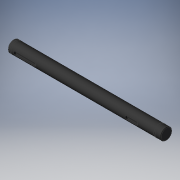
# Autodesk Inventor part: NSFMKRRA10-131-F3-S6-KA5-A19-KB100.5-B11_s
Saved by Autodesk Inventor 2019 (Build 230136000, 136)
## iProperties
Created: 2022-11-16
Part Number: NSFMKRRA10-131-F3-S6-KA5-A19-KB100.5-B11_s
Material: Generic
Catalog Web Link: www.cadenas.de
Description: NSFMKRR, SFMKRR, PSFMKRR, SSFMKRR, NSFHKRR, SFHKRR, PSFHKRR, SSFHKRR, NSFGKRR, SFGKRR, PSFGKRR, SSFGKRR, NSFMKRRA, SFMKRRA, PSFMKRRA, SSFMKRRA, NSFHKRRA, SFHKRRA, PSFHKRRA, SSFHKRRA, NSFGKRRA, SFGKRRA, PSFGKRRA, SSFGKRRA_shaft-Rotary Shafts - Retaining Ring Grooves on Both Ends with Keyway -
Vendor: MISUMI
Document SubType Name: Modeling
Designer: psAdmin
Manufacturer: MISUMI
Mass: 10.1182 g
Surface Area: 43.8116 cm^2
Volume: 10.1182 cm^3
Density: 1 g/cm^3
Appearance: PSOLRGB-175-175-175
Category: PARTsolutions
Company: MISUMI
Title: NSFMKRRA10-131-F3-S6-KA5-A19-KB100.5-B11
Author: Cadenas PARTsolutions
Comments: Rotary Shafts - Retaining Ring Grooves on Both Ends with Keyway -
PSOL_IDENT_0: {$CADENAS_DATA/23d-libs/misumi/metric/11_rotary_shafts/11_components/psfgkrr/psfgkrr.prj},638 {VTYP=
PSOL_IDENT_1: 3D},{NB=NSFMKRRA10-131-F3-S6-KA5-A19-KB100.5-B11_s},{LINA=NSFMKRRA10-131-F3-S6-KA5-A19-KB100.5-B11},
PSOL_IDENT_2: {NN=NSFMKRR, SFMKRR, PSFMKRR, SSFMKRR, NSFHKRR, SFHKRR, PSFHKRR, SSFHKRR, NSFGKRR, SFGKRR, PSFGKRR,
PSOL_IDENT_3: SSFGKRR, NSFMKRRA, SFMKRRA, PSFMKRRA, SSFMKRRA, NSFHKRRA, SFHKRRA, PSFHKRRA, SSFHKRRA, NSFGKRRA, SFG
PSOL_IDENT_4: KRRA, PSFGKRRA, SSFGKRRA_shaft},{DATE=25.01.2022 23:09:52},{GEOMDATE=05.02.2021 08:15:17},{VERSION=}
PSOL_IDENT_5: ,{LINEID=30},{WBVAR=TS,TYS,MAT,ST,ALT1,L,F,S,NOK,KA,A,KB,B,KC,C,ALT3,FC,GALT3,WFC,J,WALT3,V,ALT4,SFC
PSOL_IDENT_6: ,SG,AG,ALT10,KWC,ALT11,WC,ALT5,UC,ALT7,SC,ALT32,CD},{WBNUMERIC=L,F,S,KA,A,KB,B,KC,C,FC,GALT3,WFC,J,W
PSOL_IDENT_7: ALT3,V,SFC,SG,AG,KWC,WC,UC,SC}  {NB=NSFMKRRA10-131-F3-S6-KA5-A19-KB100.5-B11_s},{LINA=NSFMKRRA10-131
PSOL_IDENT_8: -F3-S6-KA5-A19-KB100.5-B11},{KT=DUMMY},{PN=NSFMKRRA10-131-F3-S6-KA5-A19-KB100.5-B11},{TS=A},{TSALG=''
PSOL_IDENT_9: ,'Standard','A','Retaining Ring'},{TYS=M},{TYSALG= 'M','h9 (Cold-drawn)','H','h7 (Ground)','G','g6 (
PSOL_IDENT_10: Ground)' },{MAT=S45C},{MATALG= 'S45C','S45C Equivalent', 'SUS304','304 Stainless Steel' },{ST=},{STA
PSOL_IDENT_11: LG= '','-','BO','Black Oxide', 'ENP','Electroless Nickel Plating' },{TYPE=NSFMKRR},{D=10},{ALT1=},{L
PSOL_IDENT_12: KCMAX=799.9},{L=131.0},{LALG=[15:800/0.1]},{LMIN=15},{LMAX=800},{F=3.0},{FALG=[3:126/0.1]},{FMIN=3},
PSOL_IDENT_13: {FMAX1=122.8},{FMIN2=6.2},{FMAX2=126},{S=6.0},{SALG=[3:126/0.1]},{SMIN1=3},{SMAX1=121},{SMIN2=6.2},{
PSOL_IDENT_14: SMAX2=126},{DD=9.6},{MM=1.15},{MMALG=1.2},{MMJ=2},{NOK=2},{NOKALG= '1', 'with 1 Key Groove', '2'  , '
PSOL_IDENT_15: with 2 Key Grooves', '3'  , 'with 3 Key Grooves'},{CIFNOK1=0},{CIFNOK2=3},{CIFNOK3=0},{TOL1=0},{TOL2=
PSOL_IDENT_16: 3},{TOL3=0},{BB=3},{TT=1.8},{KA=5.0},{KAALG=[5:115/0.1]},{KAMIN1=0},{KAMIN2=5},{KAMIN3=128.2},{KAMAX
PSOL_IDENT_17: 1=-1000},{KAMAX2=115},{KAMAX3=-1000},{A=19.0},{AALG=[3:100/0.1]},{AMIN=3},{AMAX=100},{AMAX1=-1000},{
PSOL_IDENT_18: AMAX2=100},{AMAX3=-1000},{KAPN=-KA5-A19},{KB=100.5},{KBALG=[26:120/0.1]},{KBMIN1=26},{KBMIN2=26},{KB
PSOL_IDENT_19: MIN3=128.2},{KBMAX1=-1000},{KBMAX2=120},{KBMAX3=-1000},{B=11.0},{BALG=[3:22.5/0.1]},{BMIN=3},{BMAX=2
PSOL_IDENT_20: 2.5},{BMAX1=-1000},{BMAX2=22.5},{BMAX3=-1000},{KBPN=-KB100.5-B11},{KC=0.0},{KCALG=[0]},{KCMIN1=113.5
PSOL_IDENT_21: },{KCMIN2=113.5},{KCMIN3=128.2},{KCMAX1=-1000},{KCMAX2=-1000},{KCMAX3=-1000},{C=0.0},{CALG=0},{CMIN=
PSOL_IDENT_22: 3},{CMAX=-1000},{CMAX1=-1000},{CMAX2=-1000},{CMAX3=-1000},{CIFKA=5},{CIFKB=3},{CIFKC=3},{KCPN=},{ALT
PSOL_IDENT_23: 3=},{ALT3ALG= '', 'w/o Set Screw Flat','FC','with FC (Adds a Set Screw Flat)','WFC','with WFC (Adds
PSOL_IDENT_24: Two Set Screw Flats)','FCWFC','with FC + WFC (Adds Three Set Screw Flats)' },{ALT3PN=},{FC=0},{FCALG=
PSOL_IDENT_25: [0]},{FCMIN=0},{FCMAX=130},{GALT3=0},{GALT3ALG=[0]},{GALT3MIN=1},{GALT3MAX=70},{GALT3MAX2=70},{GALT3
PSOL_IDENT_26: MAX3=70},{WFC=0},{WFCALG=[0]},{WFCMIN=0},{WFCMIN2=2},{WFCMAX=127},{WFCMAX2=-3},{WFCMAX3=-4},{J=0},{J
PSOL_IDENT_27: ALG=[0]},{JMIN=1},{JMAX=70},{JMAX2=-2},{JMAX3=-5},{WALT3=0},{WALT3ALG=[0]},{WALT3MIN=0},{WALT3MIN2=1
PSOL_IDENT_28: 33},{WALT3MAX=128},{WALT3MAX2=128},{V=0},{VALG=[0]},{VMIN=1},{VMAX=70},{VMAX2=70},{CIFFC=0},{ALT4=},
PSOL_IDENT_29: {ALT4ALG= '', 'w/o SFC (2 Set Screw Flats (Angle Specified))', 'SFC'  , 'with SFC (2 Set Screw Flats
PSOL_IDENT_30: (Angle Specified))'},{ALT4PN=},{SFC=0},{SFCALG=[0]},{SFCMIN=0},{SFCMAX=130},{SG=0},{SGALG=[0]},{SGM
PSOL_IDENT_31: IN=1},{SGMAX=70},{AG=0},{AGALG=[0]},{H=0},{CIFSFC=0},{ALT10=},{ALT10ALG= '','Not applicable' },{KWC=
PSOL_IDENT_32: 0},{KWCALG=[0]},{KWCMIN=1},{KWCMAX=0},{WALT10=8},{ALT10PN=},{ALT11=},{ALT11ALG= '','Not applicable'
PSOL_IDENT_33: },{WC=0.0},{WCALG=[0]},{ALT11PN=},{ALT5=},{ALT5ALG= '', 'w/o UC (Slit Cam Groove)', 'UC', 'with UC (
PSOL_IDENT_34: Slit Cam Groove)'},{ALT5PN=},{UC=0},{UCALG=[0]},{UCMIN=1},{UCMAX=125},{DDALT5=0},{LL1=0},{ALT7=},{AL
PSOL_IDENT_35: T7ALG= '', 'w/o SC (Wrench Flats)', 'SC', 'with SC (Wrench Flats)'},{ALT7PN=},{SC=0},{SCALG=[0]},{SC
PSOL_IDENT_36: MIN=0},{SCMAX=123},{LL2=0},{LL2ALG=8},{WALT7=0},{CIFSC=0},{ALT32=},{ALT32ALG= '','w/o CD (Changes Pa
PSOL_IDENT_37: rt D Chamfering)','CD','with CD (Changes Part D Chamfering)' },{CD=},{CDALG= '','N/A' },{CD3D=0.5},{
PSOL_IDENT_38: ALT32PN=},{CIF323R=0},{CIF323L=0},{CIF324R=0},{CIF324L=0},{CIF3210=0},{CIF32F=0},{CIF32S=0},{ERRORPN=
PSOL_IDENT_39: },{ERRORKGALT3=OK},{ERRORKGALT4=OK},{ERRORKGALT5=OK},{ERRORKGALT7=OK},{ERRORKGALT10=OK},{ERRORRALT3=
PSOL_IDENT_40: OK},{ERRORRALT4=NG},{ERRORRALT5=NG},{ERRORRALT7=NG},{ERRORRALT10=OK},{ERRORALT34=OK},{ERRORALT35=OK}
PSOL_IDENT_41: ,{ERRORALT37=OK},{ERRORALT310=OK},{ERRORALT45=OK},{ERRORALT47=OK},{ERRORALT410=OK},{ERRORALT57=OK},{
PSOL_IDENT_42: ERRORALT510=OK},{ERRORALT710=OK},{PCUT3D=0},{QCUT3D=0},{TTALT2=1.8},{BBALT2=3}
NB: NSFMKRRA10-131-F3-S6-KA5-A19-KB100.5-B11_s
NN: NSFMKRR, SFMKRR, PSFMKRR, SSFMKRR, NSFHKRR, SFHKRR, PSFHKRR, SSFHKRR, NSFGKRR, SFGKRR, PSFGKRR, SSFGKRR, NSFMKRRA, SFMKRRA, PSFMKRRA, SSFMKRRA, NSFHKRRA, SFHKRRA, PSFHKRRA, SSFHKRRA, NSFGKRRA, SFGKRRA, PSFGKRRA, SSFGKRRA_shaft
NT: Rotary Shafts - Retaining Ring Grooves on Both Ends with Keyway -
NBSYN: $PN._s
LINA: NSFMKRRA10-131-F3-S6-KA5-A19-KB100.5-B11
CATALOG: Misumi
PN: NSFMKRRA10-131-F3-S6-KA5-A19-KB100.5-B11
TS: Retaining Ring
TYS: h9 (Cold-drawn)
MAT: S45C Equivalent
ST: -
D: 10
ALT1: w/o LKC (Changes L Tolerance)
L: 131
F: 3
S: 6
DD: 9.6
MM: 1.15
NOK: with 2 Key Grooves
KA: 5
A: 19
KB: 100.5
B: 11
KC: 0
C: 0
ALT3: w/o Set Screw Flat
FC: 0
GALT3: 0
WFC: 0
J: 0
WALT3: 0
V: 0
ALT4: w/o SFC (2 Set Screw Flats (Angle Specified))
SFC: 0
SG: 0
AG: 0
H: 0
ALT10: Not applicable
KWC: 0
ALT11: Not applicable
WC: 0
ALT5: w/o UC (Slit Cam Groove)
UC: 0
DDALT5: 0
LL1: 0
ALT7: w/o SC (Wrench Flats)
SC: 0
LL2: 0
WALT7: 0
ALT32: w/o CD (Changes Part D Chamfering)
CD: N/A
SUPPLIER: MISUMI
ARTICLENO: NSFMKRRA10-131-F3-S6-KA5-A19-KB100.5-B11_s
BOMINFO: NSFMKRRA10-131-F3-S6-KA5-A19-KB100.5-B11
CREATOR: CADENAS GmbH
Autodesk Inventor part; units mm, degrees
sketch "Sketch_1" plane through (0, 0, 0) normal (0, 1, 0) x (-1, 0, 0)
  line L0 (-131, 0) -> (0, 0)
  line L1 (0, 0) -> (0, -4.5)
  line L2 (0, -4.5) -> (-0.5, -5)
  line L3 (-0.5, -5) -> (-130.5, -5)
  line L4 (-130.5, -5) -> (-131, -4.5)
  line L5 (-131, -4.5) -> (-131, 0)
  line L6 (-131, 0) -> (0, 0)
  constraints: 14 end point
revolve "Revolution1" add sketch "Sketch_1" angle 360 about axis through (131, 0, 0) along (1, 0, 0)
sketch "Sketch_27" plane through (0, 0, 0) normal (0, 0, 1) x (1, 0, 0)
  line L0 (131, 0) -> (-131, 0)
  line L1 (1.85, 9.6) -> (1.85, 4.8)
  line L2 (1.85, 4.8) -> (3, 4.8)
  line L3 (3, 4.8) -> (3, 9.6)
  line L4 (3, 9.6) -> (1.85, 9.6)
  constraints: 10 end point
revolve "Revolution2" cut sketch "Sketch_27" angle 360 about axis through (131, 0, 0) along (1, 0, 0)
sketch "Sketch_39" plane through (0, 0, 0) normal (0, 0, 1) x (1, 0, 0)
  line L0 (131, 0) -> (-131, 0)
  line L1 (125, 9.6) -> (125, 4.8)
  line L2 (125, 4.8) -> (126.15, 4.8)
  line L3 (126.15, 4.8) -> (126.15, 9.6)
  line L4 (126.15, 9.6) -> (125, 9.6)
  constraints: 10 end point
revolve "Revolution3" cut sketch "Sketch_39" angle 360 about axis through (131, 0, 0) along (1, 0, 0)
sketch "_____7" plane through (0, 0, 5) normal (0, 0, 1) x (1, 0, 0)
  arc A0 (6.5, 1.5) -> (6.5, -1.5) centre (6.5, 0) ccw
  line L0 (6.5, -1.5) -> (22.5, -1.5)
  arc A1 (22.5, -1.5) -> (22.5, 1.5) centre (22.5, 0) ccw
  line L1 (22.5, 1.5) -> (6.5, 1.5)
  constraints: 4 end point, 4 point on circle, 2 centre point
extrude "Extrusion1" cut sketch "_____7" against normal blind 1.8
sketch "_____10" plane through (0, 0, 5) normal (0, 0, 1) x (1, 0, 0)
  arc A0 (102, 1.5) -> (102, -1.5) centre (102, 0) ccw
  line L0 (102, -1.5) -> (110, -1.5)
  arc A1 (110, -1.5) -> (110, 1.5) centre (110, 0) ccw
  line L1 (110, 1.5) -> (102, 1.5)
  constraints: 4 end point, 4 point on circle, 2 centre point
extrude "Extrusion2" cut sketch "_____10" against normal blind 1.8
ref_plane "to_rring_1_XY" through (2.425, 0, 0) normal (1, 0, 0) x (0, 0, -1)
ref_plane "to_rring_1_YZ" through (2.425, 0, 0) normal (0, 0, -1) x (0, 1, 0)
ref_plane "to_rring_1_ZX" through (2.425, 0, 0) normal (0, 1, 0) x (1, 0, 0)
ref_plane "to_rring_2_XY" through (125.575, 0, 0) normal (1, 0, 0) x (0, 0, -1)
ref_plane "to_rring_2_YZ" through (125.575, 0, 0) normal (0, 0, -1) x (0, 1, 0)
ref_plane "to_rring_2_ZX" through (125.575, 0, 0) normal (0, 1, 0) x (1, 0, 0)
body "Solid1"
